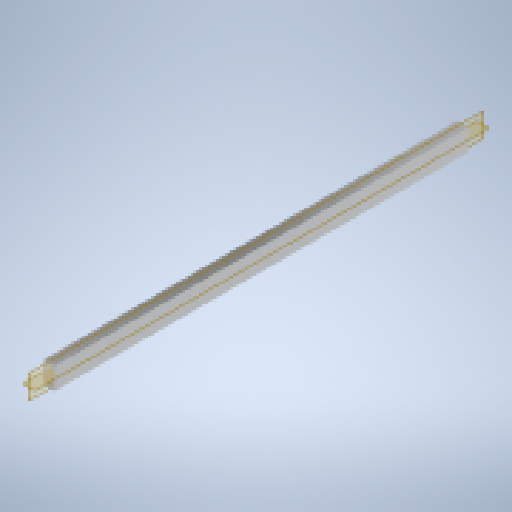
# Autodesk Inventor part: EL2-001
Saved by Autodesk Inventor 2023.4 (Build 274418000, 418)
## iProperties
RuleStatus: InUse
Created: 2025-01-10
Part Number: EL2-001
Material: Aluminum 6061
Document SubType Name: Modeling
Designer: mavericks
Mass: 304.185 g
Surface Area: 718.547 cm^2
Volume: 112.661 cm^3
Density: 2.7 g/cm^3
Appearance: Aluminum - Flat
AfterDocNew0: SHOW
AfterDocOpen0: SHOW
Author: mavericks
Autodesk Inventor part; units mm, degrees
ref_plane "XY Plane" through (0, 0, 0) normal (0, 0, 1) x (1, 0, 0)
sketch "Sketch1" plane through (0, 0, 0) normal (0, 0, 1) x (1, 0, 0)
  line L0 (-12.7, -25.4) -> (12.7, -25.4)
  line L1 (12.7, -25.4) -> (12.7, 25.4)
  line L2 (12.7, 25.4) -> (-12.7, 25.4)
  line L3 (-12.7, 25.4) -> (-12.7, -25.4)
  line L4 (-12.7, -25.4) -> (12.7, 25.4) construction
  line L5 (12.7, -25.4) -> (-12.7, 25.4) construction
  line L6 (-11.1125, 23.8125) -> (11.1125, 23.8125)
  line L7 (11.1125, 23.8125) -> (11.1125, -23.8125)
  line L8 (11.1125, -23.8125) -> (-11.1125, -23.8125)
  line L9 (-11.1125, -23.8125) -> (-11.1125, 23.8125)
  point P0 (0, 0)
  dimension "width" = 25.4
  dimension "height" = 50.8
  dimension "thickness" = 1.5875
  constraints: 20 end point, 4 parallel, 2 midpoint, 2 perpendicular, 1 horizontal, 3 other
  measures "width" distance of L2.end L1.end
  measures "height" distance of L1.end L0.end
  measures "thickness" distance between parallel lines of L2 L6
extrude "Extrusion1" add sketch "Sketch1" along normal mid plane 965.2
sketch "Sketch2" plane through (-12.7, 25.4, 482.6) normal (0, 1, 0) x (1, 0, 0)
  line L0 (0, 965.2) -> (0, 0) projected
  line L1 (0, 965.2) -> (25.4, 965.2) projected
  point P0 (12.7, 482.6)
  point P1 (12.7, 958.85)
  point P2 (12.7, 952.5)
  point P3 (12.7, 946.15)
  point P4 (12.7, 965.2)
  dimension "d5" = 12.7
  dimension "d6" = 6.35
  dimension "d7" = 6.35
  dimension "d8" = 6.35
  constraints: 2 vertical alignment, 1 midpoint
  measures "d5" distance from line of L0 point (12.7, 958.85)
  measures "d6" distance of point (12.7, 965.2) point (12.7, 958.85)
  measures "d7" distance of point (12.7, 958.85) point (12.7, 952.5)
  measures "d8" distance of point (12.7, 952.5) point (12.7, 946.15)
hole "Hole1" at (0, 25.4, -476.25) at (0, 25.4, -469.9) at (0, 25.4, -463.55) direction (0, -1, 0) diameter 5.1054 end through all clearance for "Flat Head Machine Screw (82)" size "#10" standard "Ansi Unified Screw Threads"
equation "\"d7\" = d6"
equation "\"d8\" = d6"
body "Solid1"
